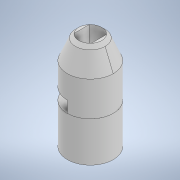
# Autodesk Inventor part: Czopek
Saved by Autodesk Inventor 2020 (Build 240168000, 168)
## iProperties
Created: 2020-04-30
Part Number: Czopek
Material: Generic
Document SubType Name: Modeling
Designer: atmat
Density: 1 g/cm^3
Appearance: Default
Author: atmat
Autodesk Inventor part; units mm, degrees
ref_plane "YZ Plane" through (0, 0, 0) normal (1, 0, 0) x (0, 1, 0)
ref_plane "XZ Plane" through (0, 0, 0) normal (0, 1, 0) x (-1, 0, 0)
ref_plane "XY Plane" through (0, 0, 0) normal (0, 0, 1) x (1, 0, 0)
sketch "Sketch1" plane through (0, 0, 0) normal (0, 1, 0) x (-1, 0, 0)
  circle A0 centre (0, 0) radius 4
  dimension "d0" = 8
  constraints: 1 centre point, 1 coincident
  measures "d0" diameter of A0
extrude "Extrusion1" add sketch "Sketch1" along normal blind 7
sketch "Sketch2" plane through (0, 7, 0) normal (0, 1, 0) x (1, 0, 0)
  circle A0 centre (0, 0) radius 4
  constraints: 1 centre point, 1 coincident
extrude "Extrusion2" add sketch "Sketch2" along normal blind 10 separate body
sketch "Sketch3" plane through (0, 17, 0) normal (0, 1, 0) x (1, 0, 0)
  line L0 (-1.5, -1.3229) -> (1.5, -1.3229)
  line L1 (1.5, -1.3229) -> (1.5, 1.3229)
  line L2 (1.5, 1.3229) -> (-1.5, 1.3229)
  line L3 (-1.5, 1.3229) -> (-1.5, -1.3229)
  circle A0 centre (0, 0) radius 2
  point P0 (-1.5, 1.3229)
  dimension "d5" = 3
  dimension "d6" = 4
  constraints: 8 end point, 3 point on circle, 2 parallel, 1 centre point, 1 coincident, 1 horizontal, 1 perpendicular
  measures "d5" distance between parallel lines of L1 L3
  measures "d6" diameter of A0
extrude "Extrusion3" cut sketch "Sketch3" against normal blind 7 contours L3 L2 L1 L0 | L0 A0 | A0 L2 bodies 1 2
chamfer "Chamfer1" distance 2 angle 45 1 edges at (-4, 17, 0)
chamfer "Chamfer2" distance 2 angle 45 1 edges at (-4, 15.0005, 0)
sketch "Sketch4" plane through (0, 0, 0) normal (1, 0, 0) x (0, 1, 0)
  line L0 (7, -4) -> (7, 4) projected
  line L1 (7, 4) -> (13, 4) projected
  line L2 (7, -4) -> (9, -4)
  line L3 (9, -4) -> (9, 4)
  line L4 (9, 4) -> (7, 4)
  line L5 (7, 4) -> (7, -4)
  point P0 (0, 0)
  dimension "d15" = 2
  constraints: 8 end point, 2 parallel, 1 horizontal, 1 perpendicular, 1 point on line
  measures "d15" distance between parallel lines of L0 L3
extrude "Extrusion4" cut sketch "Sketch4" against normal blind 7 bodies 1 2
body "Solid1"
body "Solid3"
